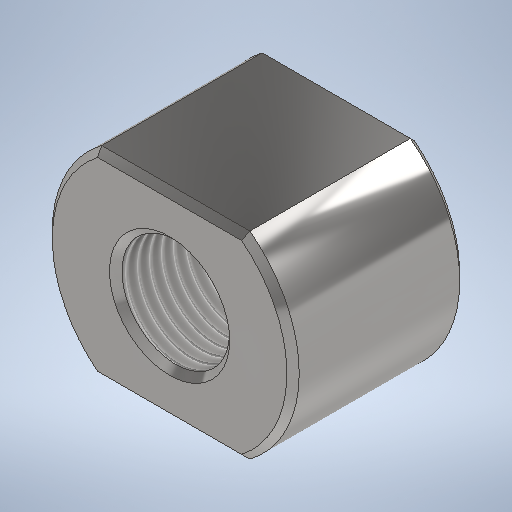
# Autodesk Inventor part: NozzleConnector
Saved by Autodesk Inventor 2025.2 (Build 292293000, 293)
## iProperties
Created: 2026-07-22
Part Number: NozzleConnector
Material: Generic
Document SubType Name: Modeling
Designer: Simon
Density: 1 g/cm^3
Appearance: Steel - Polished
Author: Simon
Autodesk Inventor part; units mm, degrees
ref_plane "YZ Plane" through (0, 0, 0) normal (1, 0, 0) x (0, 1, 0)
ref_plane "XZ Plane" through (0, 0, 0) normal (0, 1, 0) x (-1, 0, 0)
ref_plane "XY Plane" through (0, 0, 0) normal (0, 0, 1) x (1, 0, 0)
sketch "Sketch1" plane through (0, 0, 0) normal (0, 0, 1) x (1, 0, 0)
  circle A0 centre (0, 0) radius 10
  line L0 (0, 10) -> (0, 8)
  line L1 (0, -10) -> (0, -8)
  line L2 (-6, -8) -> (6, -8)
  line L3 (-6, 8) -> (6, 8)
  point P0 (-6, 8)
  point P1 (-6, -8)
  dimension "d0" = 20
  dimension "d28" = 2
  dimension "d29" = 2
  constraints: 8 end point, 4 point on circle, 2 midpoint, 2 vertical, 1 centre point, 1 coincident, 1 horizontal, 1 parallel
  measures "d0" diameter of A0
  measures "d28" distance of L0.start L0.end
  measures "d29" distance of L1.start L1.end
extrude "Extrusion1" add sketch "Sketch1" against normal blind 14 contours A0 L2 L3
hole "Hole1" at (0, 0, 0) direction (0, 0, -1) diameter 7.9502 depth 7 taper from width 8.7366 to width 8.304 over 6.924 thread size "1/8" designation "1/8 - 27 NPT" standard "NPT"
hole "Hole2" at (0, 0, 0) direction (0, 0, -1) diameter 6 end through all
thread "Thread2" size "M6x1" class "6H" standard "ANSI Metric M Profile" length 7
chamfer "Chamfer3" distance 0.5 angle 45 8 edges at (0, 8, 0) (0, -8, 0) (10, 0, 0) (-10, 0, 0) (0, -8, -14) (0, 8, -14) (10, 0, -14) (-10, 0, -14)
chamfer "Chamfer4" distance 0.5 angle 45 2 edges at (0, 4.3683, 0) (0, 3, -14)
body "Solid1"
